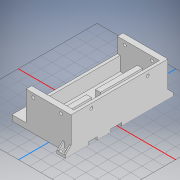
# Autodesk Inventor part: 000.003.001 - Основание
Saved by Autodesk Inventor 2022 (Build 260153000, 153)
## iProperties
Created: 2022-02-26
Part Number: 000.003.001 - Основание
Material: Типовые
Document SubType Name: Modeling
Designer: Petrov Ivan
Density: 1 g/cm^3
Appearance: По умолчанию
Author: Petrov Ivan
Autodesk Inventor part; units mm, degrees
ref_plane "YZ Plane" through (0, 0, 0) normal (1, 0, 0) x (0, 1, 0)
ref_plane "XZ Plane" through (0, 0, 0) normal (0, 1, 0) x (-1, 0, 0)
ref_plane "XY Plane" through (0, 0, 0) normal (0, 0, 1) x (1, 0, 0)
sketch "Эскиз1" plane through (0, 0, 0) normal (0, 1, 0) x (-1, 0, 0)
  line L0 (40, 86.25) -> (-40, 86.25)
  line L1 (-40, 86.25) -> (-40, -86.25)
  line L2 (-40, -86.25) -> (40, -86.25)
  line L3 (40, -86.25) -> (40, 86.25)
  point P0 (0, 0)
  dimension "d0" = 80
  dimension "d1" = 172.5
  dimension "d29" = 86.25
  dimension "d30" = 40
  constraints: 8 end point, 2 parallel, 1 horizontal, 1 perpendicular
  measures "d0" distance of L2.end L1.end
  measures "d1" distance of L1.end L0.end
  measures "d29" distance from line of point (0, 0) L2
  measures "d30" distance from line of point (0, 0) L1
extrude "Выдавливание1" add sketch "Эскиз1" along normal blind 10
sketch "Эскиз3" plane through (0, 10, 0) normal (0, 1, 0) x (1, 0, 0)
  line L0 (-40, 86.25) -> (-40, -86.25) projected
  line L1 (-40, 86.25) -> (-40, 76.25)
  line L2 (-40, 76.25) -> (35, 76.25)
  line L3 (35, 76.25) -> (35, -76.25)
  line L4 (35, -76.25) -> (-40, -76.25)
  line L5 (-40, -86.25) -> (40, -86.25) projected
  line L6 (40, 86.25) -> (-40, 86.25) projected
  line L7 (40, -86.25) -> (40, 86.25) projected
  point P0 (0, 0)
  point P1 (-40, -76.25)
  dimension "d11" = 10
  dimension "d12" = 10
  dimension "d13" = 5
  constraints: 8 end point, 2 perpendicular, 2 point on line, 1 horizontal
  measures "d11" distance between parallel lines of L4 L5
  measures "d12" distance between parallel lines of L6 L2
  measures "d13" distance between parallel lines of L7 L3
extrude "Выдавливание3" add sketch "Эскиз3" along normal blind 52 contours L6 L7 L5 L0 L4 L3 L2
sketch "Эскиз4" plane through (0, 0, 0) normal (0, -1, 0) x (1, 0, 0)
  line L0 (-40, 86.25) -> (40, 86.25) projected
  line L1 (40, 86.25) -> (25, 86.25)
  line L2 (25, 86.25) -> (25, 96.25)
  line L3 (25, 96.25) -> (40, 96.25)
  line L4 (40, 96.25) -> (40, 86.25)
  circle A0 centre (32.5, 91.25) radius 2.775
  point P0 (0, 0)
  point P1 (32.5, 96.25)
  dimension "d16" = 15
  dimension "d17" = 10
  dimension "d18" = 5.55
  constraints: 8 end point, 2 parallel, 1 centre point, 1 horizontal, 1 midpoint, 1 perpendicular, 1 vertical alignment
  measures "d16" distance of L2.end L3.end
  measures "d17" distance of L1.end L2.end
  measures "d18" diameter of A0
extrude "Выдавливание4" add sketch "Эскиз4" against normal blind 5
sketch "Эскиз5" plane through (0, 5, 0) normal (0, 1, 0) x (1, 0, 0)
  line L0 (25, -86.25) -> (25, -96.25) projected
  line L1 (-40, -86.25) -> (40, -86.25) projected
  line L2 (25, -96.25) -> (27.5, -96.25)
  line L3 (27.5, -96.25) -> (27.5, -86.25)
  line L4 (27.5, -86.25) -> (25, -86.25)
  line L5 (25, -86.25) -> (25, -96.25)
  line L6 (40, -96.25) -> (40, 86.25) projected
  line L7 (40, -96.25) -> (37.5, -96.25)
  line L8 (37.5, -96.25) -> (37.5, -86.25)
  line L9 (37.5, -86.25) -> (40, -86.25)
  line L10 (40, -86.25) -> (40, -96.25)
  point P0 (0, 0)
  dimension "d21" = 2.5
  dimension "d22" = 2.5
  constraints: 16 end point, 4 parallel, 2 horizontal, 2 perpendicular, 2 point on line
  measures "d21" distance between parallel lines of L0 L3
  measures "d22" distance between parallel lines of L6 L8
extrude "Выдавливание5" add sketch "Эскиз5" along normal blind 10
chamfer "Фаска1" distance 10 angle 45 2 edges at (26.25, 15, 96.25) (38.75, 15, 96.25)
mirror "Зеркальное отражение3" about plane through (0, 0, 0) normal (0, 0, 1) of "Выдавливание4", "Выдавливание5", "Фаска1"
sketch "Эскиз6" plane through (-40, 0, -86.25) normal (-1, 0, 0) x (0, 0, 1)
  line L0 (172.5, 0) -> (172.5, 15) projected
  line L1 (0, 0) -> (0, 62) projected
  line L2 (172.5, 10) -> (0, 10)
  line L3 (0, 10) -> (0, 0)
  line L4 (0, 0) -> (172.5, 0)
  line L5 (172.5, 0) -> (172.5, 10)
  point P0 (86.25, 0)
  point P1 (10, 10)
  point P2 (0, 10)
  constraints: 8 end point, 2 parallel, 2 point on line, 1 horizontal, 1 perpendicular
extrude "Выдавливание6" add sketch "Эскиз6" along normal blind 25
sketch "Эскиз8" plane through (-40, 62, 86.25) normal (0, 0, 1) x (1, 0, 0)
  circle A0 centre (13, -7) radius 2.75
  circle A1 centre (62, -7) radius 2.75
  line L0 (75, -52) -> (75, 0) projected
  line L1 (77.5, -47) -> (80, -47) projected
  line L2 (80, -47) -> (80, 0) projected
  line L3 (0, 0) -> (80, 0) projected
  line L4 (0, -52) -> (0, 0) projected
  line L5 (65, -62) -> (65, -47) projected
  line L6 (65, -47) -> (67.5, -47) projected
  line L7 (67.5, -47) -> (67.5, -57) projected
  line L8 (67.5, -57) -> (77.5, -57) projected
  line L9 (77.5, -57) -> (77.5, -47) projected
  line L10 (65, -62) -> (-25, -62) projected
  line L11 (0, -52) -> (-25, -52) projected
  line L12 (-25, -62) -> (-25, -52) projected
  point P0 (40, -62)
  dimension "d37" = 5.5
  dimension "d38" = 5.5
  dimension "d39" = 7
  dimension "d40" = 13
  dimension "d41" = 13
  constraints: 2 centre point, 1 horizontal alignment
  measures "d37" diameter of A0
  measures "d38" diameter of A1
  measures "d39" distance from line of L3 A1.centre
  measures "d40" distance from line of L0 A1.centre
  measures "d41" distance from line of L4 A0.centre
extrude "Выдавливание8" cut sketch "Эскиз8" against normal through all contours A0 | A1
sketch "Эскиз9" plane through (40, 62, 86.25) normal (1, 0, 0) x (0, 0, -1)
  circle A0 centre (36.25, -8) radius 2.75
  circle A1 centre (136.25, -8) radius 2.75
  line L0 (0, 0) -> (172.5, 0) projected
  line L1 (162.5, 0) -> (10, 0) projected
  line L2 (86.25, 0) -> (86.25, -11.5719) construction
  point P0 (86.25, -62)
  dimension "d44" = 5.5
  dimension "d45" = 5.5
  dimension "d46" = 8
  dimension "d50" = 50
  constraints: 2 centre point, 2 end point, 1 horizontal alignment, 1 midpoint, 1 symmetric about line, 1 vertical
  measures "d44" diameter of A0
  measures "d45" diameter of A1
  measures "d46" distance from line of L0 A0.centre
  measures "d50" distance from line of L2 A0.centre
extrude "Выдавливание9" cut sketch "Эскиз9" against normal blind 10
sketch "Эскиз10" plane through (0, 10, 0) normal (0, 1, 0) x (1, 0, 0)
  line L0 (25, -23.75) -> (12.5, -23.75)
  line L1 (12.5, -23.75) -> (12.5, -29.75)
  line L2 (12.5, -29.75) -> (25, -29.75)
  line L3 (-25, -23.75) -> (-12.5, -23.75)
  line L4 (-12.5, -23.75) -> (-12.5, -29.75)
  line L5 (-12.5, -29.75) -> (-25, -29.75)
  line L6 (-25, -29.75) -> (-25, -23.75)
  line L7 (25, -29.75) -> (25, -23.75)
  line L8 (35, 76.25) -> (35, -76.25) projected
  line L9 (-40, 76.25) -> (35, 76.25) projected
  point P0 (0, 0)
  dimension "d51" = 12.5
  dimension "d52" = 6
  dimension "d53" = 12.5
  dimension "d54" = 6
  dimension "d55" = 25
  dimension "d56" = 10
  dimension "d59" = 100
  dimension "d60" = 100
  constraints: 16 end point, 3 parallel, 3 perpendicular, 2 horizontal
  measures "d51" distance of L1.end L2.end
  measures "d52" distance of L0.end L1.end
  measures "d53" distance of L4.end L5.end
  measures "d54" distance of L3.end L4.end
  measures "d55" distance between parallel lines of L1 L4
  measures "d56" distance between parallel lines of L8 L7
  measures "d59" distance between parallel lines of L9 L0
  measures "d60" distance between parallel lines of L9 L3
extrude "Выдавливание10" cut sketch "Эскиз10" against normal through all
sketch "Эскиз11" plane through (0, 0, 0) normal (0, -1, 0) x (1, 0, 0)
  line L0 (25, 29.75) -> (12.5, 29.75)
  line L1 (12.5, 29.75) -> (12.5, 39.75)
  line L2 (12.5, 39.75) -> (25, 39.75)
  line L3 (25, 39.75) -> (25, 29.75)
  line L4 (-12.5, 29.75) -> (-25, 29.75) projected
  line L5 (-12.5, 29.75) -> (-25, 29.75)
  line L6 (-25, 29.75) -> (-25, 39.75)
  line L7 (-25, 39.75) -> (-12.5, 39.75)
  line L8 (-12.5, 39.75) -> (-12.5, 29.75)
  line L9 (40, 96.25) -> (40, -96.25) projected
  line L10 (-25, 39.75) -> (40, 39.75)
  line L11 (40, 39.75) -> (40, 54.75)
  line L12 (40, 54.75) -> (-25, 54.75)
  line L13 (-25, 54.75) -> (-25, 39.75)
  point P0 (0, 0)
  point P1 (-25, 29.75)
  point P2 (-12.5, 39.75)
  point P3 (12.5, 39.75)
  point P4 (25, 39.75)
  point P5 (40, 39.75)
  dimension "d61" = 10
  dimension "d62" = 15
  dimension "d63" = 12.5
  constraints: 24 end point, 6 parallel, 3 horizontal, 3 perpendicular, 2 point on line
  measures "d61" distance of L0.end L1.end
  measures "d62" distance between parallel lines of L12 L10
  measures "d63" distance between parallel lines of L6 L8
extrude "Выдавливание11" cut sketch "Эскиз11" against normal blind 5
sketch "Эскиз12" plane through (0, 10, 0) normal (0, 1, 0) x (1, 0, 0)
  line L0 (35, -76.25) -> (-40, -76.25) projected
  line L1 (35, 76.25) -> (-40, 76.25) projected
  line L2 (-4.5, -76.25) -> (4.5, -76.25)
  line L3 (4.5, -76.25) -> (4.5, 76.25)
  line L4 (4.5, 76.25) -> (-4.5, 76.25)
  line L5 (-4.5, 76.25) -> (-4.5, -76.25)
  line L6 (-12.5, -23.75) -> (-12.5, -29.75) projected
  line L7 (12.5, -29.75) -> (12.5, -23.75) projected
  point P0 (0, 0)
  dimension "d66" = 8
  dimension "d67" = 8
  constraints: 8 end point, 2 parallel, 2 point on line, 1 horizontal, 1 perpendicular
  measures "d66" distance between parallel lines of L6 L5
  measures "d67" distance between parallel lines of L7 L3
extrude "Выдавливание12" add sketch "Эскиз12" along normal blind 25
sketch "Эскиз13" plane through (0, 10, 0) normal (0, 1, 0) x (1, 0, 0)
  line L0 (-40, 86.25) -> (-40, 76.25) projected
  line L1 (35, -76.25) -> (-40, -76.25) projected
  line L2 (-40, 76.25) -> (-35, 76.25)
  line L3 (-35, 76.25) -> (-35, -76.25)
  line L4 (-35, -76.25) -> (-40, -76.25)
  line L5 (-40, -76.25) -> (-40, 76.25)
  point P0 (0, 0)
  dimension "d70" = 5
  constraints: 8 end point, 2 parallel, 1 horizontal, 1 perpendicular, 1 point on line
  measures "d70" distance between parallel lines of L5 L3
extrude "Выдавливание13" add sketch "Эскиз13" along normal up to surface (25 mm away)
sketch "Эскиз15" plane through (0, 35, 0) normal (0, 1, 0) x (1, 0, 0)
  line L0 (4.5, 76.25) -> (4.5, -76.25) projected
  line L1 (-4.5, 1.75) -> (4.5, 1.75)
  line L2 (4.5, 1.75) -> (4.5, -14.25)
  line L3 (4.5, -14.25) -> (-4.5, -14.25)
  line L4 (-4.5, -14.25) -> (-4.5, 1.75)
  line L5 (-4.5, 1.75) -> (4.5, -14.25) construction
  line L6 (4.5, 1.75) -> (-4.5, -14.25) construction
  line L7 (-7.5, -14.25) -> (7.5, -14.25)
  line L8 (7.5, -14.25) -> (7.5, 1.75)
  line L9 (7.5, 1.75) -> (-7.5, 1.75)
  line L10 (-7.5, 1.75) -> (-7.5, -14.25)
  line L11 (-7.5, -14.25) -> (7.5, 1.75) construction
  line L12 (7.5, -14.25) -> (-7.5, 1.75) construction
  line L13 (35, -76.25) -> (-40, -76.25) projected
  point P0 (0, -6.25)
  point P1 (4.5, 1.75)
  point P2 (4.5, 1.75)
  point P3 (4.5, -14.25)
  point P4 (-4.5, -14.25)
  point P5 (-4.5, 1.75)
  point P6 (0, -6.25)
  dimension "d76" = 16
  dimension "d83" = 15
  dimension "d84" = 70
  dimension "d85" = 16
  constraints: 24 end point, 5 midpoint, 4 parallel, 2 horizontal, 2 perpendicular, 1 point on line
  measures "d76" distance of L1.end L2.end
  measures "d83" distance of L9.end L8.end
  measures "d84" distance from line of L13 point (0, -6.25)
  measures "d85" distance of L7.end L8.end
extrude "Выдавливание15" cut sketch "Эскиз15" against normal through all
sketch "Эскиз17" plane through (0, 0, 0) normal (0, -1, 0) x (1, 0, 0)
  line L0 (21.6513, 14.3273) -> (57.2013, 14.3235) projected
  line L1 (21.6521, 22.2773) -> (21.6513, 14.3273) projected
  line L2 (11.4921, 22.2784) -> (21.6521, 22.2773) projected
  line L3 (11.4913, 14.3314) -> (11.4921, 22.2784) projected
  line L4 (-16.4487, 14.3314) -> (11.4913, 14.3314) projected
  line L5 (-16.4506, -3.1186) -> (-16.4487, 14.3314) projected
  line L6 (11.4894, -3.1216) -> (-16.4506, -3.1186) projected
  line L7 (11.4884, -12.0116) -> (11.4894, -3.1216) projected
  line L8 (21.6484, -12.0127) -> (11.4884, -12.0116) projected
  line L9 (21.6494, -3.1227) -> (21.6484, -12.0127) projected
  line L10 (57.1994, -3.1265) -> (21.6494, -3.1227) projected
  line L11 (57.2013, 14.3235) -> (57.1994, -3.1265) projected
  circle A0 centre (17.2067, 18.5947) radius 1.5 projected
  circle A1 centre (17.0769, -7.8212) radius 1.5 projected
  circle A2 centre (-12.6397, 5.771) radius 1.5 projected
  point P0 (0, 0)
ref_plane "РабПлоскость1" through (-7.5, 9.111, -1.6) normal (0, -1, 0) x (1, 0, 0)
extrude "Выдавливание17" cut sketch "Эскиз17" against normal blind 5 contours L0 L11 L10 L9 L8 L7 L6 L5 L4 L3 L2 L1 | A0 | A1 | A2
offset faces "Размер1" outward -1 faces at (27.7675, 3.3333, 14.3266) (21.6515, 1.6667, 16.9773) (18.2654, 1.6667, 22.2776) (11.4918, 1.6667, 19.6294) (2.1779, 3.3333, 14.3314) (-16.4494, 1.6667, 8.5147) (-7.1373, 1.6667, -3.1196) (14.8751, 1.6667, -12.012) (33.8831, 3.3333, -3.124) (11.4891, 1.6667, -6.085) (21.6487, 1.6667, -9.0494)
sketch "Эскиз18" plane through (-17.4486, 5, 15.3314) normal (0, -1, 0) x (1, 0, 0)
  circle A0 centre (34.6554, 3.2634) radius 1.5 projected
  circle A1 centre (34.5255, -23.1526) radius 1.5 projected
  circle A2 centre (4.809, -9.5604) radius 1.5 projected
  point P0 (17.4486, -15.3314)
extrude "Выдавливание18" cut sketch "Эскиз18" against normal blind 5
offset faces "Размер2" outward -0.5 faces at (18.6873, 8.3333, 18.3541) (18.5575, 8.3333, -8.0619) (-11.1591, 8.3333, 5.5303)
sketch "Эскиз19" plane through (0, 10, 0) normal (0, 1, 0) x (1, 0, 0)
  circle A0 centre (-56, 56) radius 1.85 projected
  circle A1 centre (-56, -56) radius 1.85 projected
  point P0 (0, 0)
extrude "Выдавливание19" cut sketch "Эскиз19" against normal through all
offset faces "Размер3" outward -0.25 faces at (19.1808, 8.3333, 18.2739) (19.051, 8.3333, -8.1421) (-10.6656, 8.3333, 5.4501)
equation "\"d29\" = 0.5 * d1"
equation "\"d30\" = 0.5 * d0"
equation "\"d12\" = d11"
equation "\"d59\" = d60"
equation "\"d67\" = d66"
